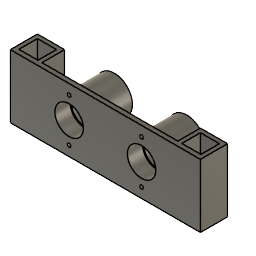
pump_holder_EZO-PMP (Autodesk Fusion 360 design; units mm, degrees)
Autodesk Fusion 360 part; units mm, degrees
sketch "Sketch1" plane through (0, 0, 0) normal (0, 0, 1) x (1, 0, 0)
  line L0 (0, 0) -> (210, 0)
  line L1 (210, 0) -> (210, 5)
  line L2 (210, 5) -> (0, 5)
  line L3 (0, 5) -> (0, 0)
  line L4 (0, 0) -> (30, 0)
  line L5 (30, 0) -> (30, 30)
  line L6 (30, 30) -> (0, 30)
  line L7 (0, 30) -> (0, 0)
  line L8 (4.5, 25.5) -> (25.5, 25.5)
  line L9 (25.5, 25.5) -> (25.5, 5)
  line L10 (25.5, 5) -> (4.5, 5)
  line L11 (4.5, 5) -> (4.5, 25.5)
  line L12 (210, 0) -> (180, 0)
  line L13 (180, 0) -> (180, 30)
  line L14 (180, 30) -> (210, 30)
  line L15 (210, 30) -> (210, 0)
  line L16 (205.5, 5) -> (184.5, 5)
  line L17 (184.5, 5) -> (205.5, 5)
  line L18 (205.5, 5) -> (205.5, 25.5)
  line L19 (205.5, 25.5) -> (184.5, 25.5)
  line L20 (184.5, 25.5) -> (184.5, 5)
  dimension "d1" = 210
  dimension "d2" = 5
  dimension "d3" = 30
  dimension "d4" = 30
  dimension "d9" = 21
  dimension "d75" = 4.5
  dimension "d76" = 4.5
  dimension "d77" = 4.5
  dimension "d78" = 4.5
  dimension "d79" = 4.5
  constraint horizontal L0
  constraint vertical L1
  constraint horizontal L2
  constraint vertical L3
  constraint coincident L0.start L3.end
  constraint horizontal L4
  constraint vertical L5
  constraint horizontal L6
  constraint vertical L7
  constraint horizontal L8
  constraint vertical L9
  constraint horizontal L10
  constraint vertical L11
  constraint coincident L2 L9.end
  constraint horizontal L12
  constraint vertical L13
  constraint horizontal L14
  constraint vertical L15
  constraint horizontal L16
  constraint coincident L2 L16.start
  constraint horizontal L17
  constraint vertical L18
  constraint horizontal L19
  constraint vertical L20
  measures "d1" distance of L0.start L0.end
  measures "d2" distance of L0.start L2.end
  measures "d3" distance of L5.end L6.end
  measures "d4" distance of L4.end L5.end
  measures "d9" distance of L16.start L16.end
  measures "d75" distance of L15 L18
  measures "d76" distance of L14 L19
  measures "d77" distance of L5 L9
  measures "d78" distance of L7 L11
  measures "d79" distance of L6 L8
extrude "Extrude1" add sketch "Sketch1" along normal blind 70 contours L0 L2 L3 L4 L5 L7 L10 | L0 L2 L5 L13 | L2 L5 L6 L7 L8 L9 L11 | L0 L1 L2 L12 L13 L15 L16 L17 | L2 L13 L14 L15 L18 L19 L20 | L2 L16 L17 L18 L19 L20 makes body 1
sketch "Sketch2" plane through (0, 5, 0) normal (0, 1, 0) x (-1, 0, 0)
  line L0 (-180, 0) -> (-30, 0)
  line L1 (-30, 0) -> (-30, 70)
  line L2 (-30, 70) -> (-180, 70)
  line L3 (-180, 70) -> (-180, 0)
  circle A0 centre (-65, 35) radius 15.75
  circle A1 centre (-145, 35) radius 15.75
  line L4 (-105, 0) -> (-105, 70)
  circle A2 centre (-145, 35) radius 20
  circle A3 centre (-65, 35) radius 20
  circle A4 centre (-65, 11) radius 2
  circle A5 centre (-65, 59) radius 2
  circle A6 centre (-145, 59) radius 2
  circle A7 centre (-145, 11) radius 2
  circle A8 centre (-65, 35) radius 14.25
  circle A9 centre (-145, 35) radius 14.25
  dimension "d14" = 105
  dimension "d15" = 40
  dimension "d16" = 40
  dimension "d17" = 31.5
  dimension "d18" = 31.5
  dimension "d20" = 40
  dimension "d21" = 40
  dimension "d26" = 35
  dimension "d27" = 35
  dimension "d28" = 24
  dimension "d29" = 24
  dimension "d30" = 24
  dimension "d31" = 24
  dimension "d32" = 4
  dimension "d33" = 4
  dimension "d34" = 4
  dimension "d35" = 4
  dimension "d36" = 40
  dimension "d37" = 40
  dimension "d38" = 40
  dimension "d39" = 40
  dimension "d42" = 28.5
  dimension "d43" = 28.5
  constraint coincident L0 L4.start
  constraint coincident L2 L4.end
  constraint perpendicular L2 L4
  constraint concentric A1 A2
  constraint concentric A0 A3
  constraint concentric A0 A8
  constraint concentric A2 A9
  measures "d14" distance of origin L4
  measures "d15" distance of A1.centre L4
  measures "d16" distance of A0.centre L4
  measures "d17" diameter of A0
  measures "d18" diameter of A1
  measures "d20" diameter of A3
  measures "d21" diameter of A2
  measures "d26" distance of L0 A0.centre
  measures "d27" distance of L0 A1.centre
  measures "d28" vertical distance of A0.centre A4.centre
  measures "d29" vertical distance of A0.centre A5.centre
  measures "d30" vertical distance of A1.centre A6.centre
  measures "d31" vertical distance of A1.centre A7.centre
  measures "d32" diameter of A5
  measures "d33" diameter of A4
  measures "d34" diameter of A7
  measures "d35" diameter of A6
  measures "d36" distance of L4 A7.centre
  measures "d37" distance of L4 A6.centre
  measures "d38" distance of L4 A5.centre
  measures "d39" distance of L4 A4.centre
  measures "d42" diameter of A8
  measures "d43" diameter of A9
extrude "Extrude2" cut sketch "Sketch2" against normal blind 140 contours A0 | A1 | A8 | A9 bodies 1
extrude "Extrude3" add sketch "Sketch2" along normal blind 45 contours A2 | A3 bodies 1
extrude "Extrude4" cut sketch "Sketch2" against normal blind 31 contours A4 | A5 | A6 | A7 bodies 1
extrude "Extrude5" add sketch "Sketch2" along normal blind 33 contours A0 | A1 bodies 1
delete_face "DeleteFace1" 1 faces at (130.0949, 38, 38.0379) on bodies 1
delete_face "DeleteFace2" 1 faces at (49.8617, 38, 33.5096) on bodies 1
extrude "Extrude6" add sketch "Sketch2" along normal blind 33 contours A0 | A1 bodies 1
delete_face "DeleteFace3" 1 faces at (49.8617, 38, 33.5096) on bodies 1
delete_face "DeleteFace4" 1 faces at (130.0949, 38, 38.0379) on bodies 1
extrude "Extrude7" cut sketch "Sketch2" against normal blind 5 contours A4 | A5 | A6 | A7 | A8 | A9 bodies 1
extrude "Extrude8" add sketch "Sketch2" along normal blind 33 contours A0 | A1 bodies 1
delete_face "DeleteFace5" 1 faces at (49.8617, 38, 33.5096) on bodies 1
delete_face "DeleteFace6" 1 faces at (130.0949, 38, 38.0379) on bodies 1
sketch "Sketch3" plane through (0, 30, 0) normal (0, 1, 0) x (-1, 0, 0)
  line L0 (-210, 0) -> (-180, 0)
  line L1 (-180, 0) -> (-180, 70)
  line L2 (-180, 70) -> (-210, 70)
  line L3 (-210, 70) -> (-210, 0)
  circle A0 centre (-195, 35) radius 4.75
  circle A1 centre (-15, 35) radius 4.75
  line L4 (-30, 70) -> (0, 70)
  line L5 (0, 0) -> (0, 70)
  circle A2 centre (-15, 35) radius 2.75
  circle A3 centre (-195, 35) radius 2.75
  dimension "d54" = 35
  dimension "d55" = 15
  dimension "d56" = 9.5
  dimension "d57" = 35
  dimension "d58" = 15
  dimension "d59" = 9.5
  dimension "d61" = 5.5
  dimension "d74" = 5.5
  constraint concentric A1 A2
  constraint concentric A0 A3
  measures "d54" distance of L2 A0.centre
  measures "d55" distance of L3 A0.centre
  measures "d56" diameter of A0
  measures "d57" distance of A1.centre L4
  measures "d58" distance of A1.centre L5
  measures "d59" diameter of A1
  measures "d61" diameter of A2
  measures "d74" diameter of A3
extrude "Extrude19" cut sketch "Sketch3" against normal blind 5 contours A0 | A3 bodies 1
extrude "Extrude20" cut sketch "Sketch1" along normal blind 100 contours L2 L16 L17 L18 L19 L20 bodies 1
extrude "Extrude21" cut sketch "Sketch3" against normal blind 5 contours A1 | A2 bodies 1
extrude "Extrude22" add sketch "Sketch3" along normal blind 2.5 separate body contours A1 makes body 2
extrude "Extrude23" add sketch "Sketch3" along normal blind 2.5 separate body contours A0 makes body 3
move_body "Move4" bodies 3 to x (1, 0, 0) y (0, 1, 0) z (0, 0, 1) at (0, -4.5, 0)
move_body "Move5" bodies 2 to x (1, 0, 0) y (0, 1, 0) z (0, 0, 1) at (0, -4.5, 0)
extrude "Extrude24" add sketch "Sketch2" along normal blind 33 separate body contours A1 makes body 4
extrude "Extrude25" add sketch "Sketch2" along normal blind 33 separate body contours A0 makes body 5
move_body "Move6" bodies 5 to x (1, 0, 0) y (0, 1, 0) z (0, 0, 1) at (0, 12, 0)
move_body "Move7" bodies 4 to x (1, 0, 0) y (0, 1, 0) z (0, 0, 1) at (0, 12, 0)
extrude "Extrude10" cut sketch "Sketch3" against normal blind 5 contours A1 | A2 bodies 1
extrude "Extrude11" [suppressed]
extrude "Extrude12" [suppressed]
extrude "Extrude13" [suppressed]
extrude "Extrude14" [suppressed]
extrude "Extrude15" [suppressed]
move_body "Move2" [suppressed]
extrude "Extrude16" [suppressed]
extrude "Extrude17" [suppressed]
extrude "Extrude18" [suppressed]
move_body "Move3" [suppressed]
